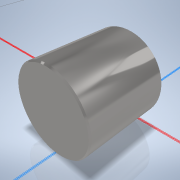
# Autodesk Inventor part: ciezarek
Saved by Autodesk Inventor 2021 (Build 250183000, 183)
## iProperties
Created: 2021-11-16
Part Number: ciezarek
Material: Stal nierdzewna 440C
Document SubType Name: Modeling
Designer: wojwo
Mass: 48.6178 g
Surface Area: 18.5509 cm^2
Volume: 6.27327 cm^3
Density: 7.75 g/cm^3
Appearance: Częściowo polerowana
Author: wojwo
Autodesk Inventor part; units mm, degrees
ref_plane "YZ Plane" through (0, 0, 0) normal (1, 0, 0) x (0, 1, 0)
ref_plane "XZ Plane" through (0, 0, 0) normal (0, 1, 0) x (-1, 0, 0)
ref_plane "XY Plane" through (0, 0, 0) normal (0, 0, 1) x (1, 0, 0)
sketch "Szkic1" plane through (0, 0, 0) normal (0, 0, 1) x (1, 0, 0)
  circle A0 centre (0, -7.5) radius 4.5 projected
  circle A1 centre (0, 0) radius 39.6 projected
  circle A2 centre (0, 7.5) radius 4.5 projected
  circle A3 centre (0, -7.5) radius 4.5 projected
  circle A4 centre (0, 0) radius 39.6 projected
  circle A5 centre (0, 7.5) radius 4.5 projected
  circle A6 centre (0, 20) radius 10
  point P0 (0, 0)
  dimension "d0" = 20
  dimension "d6" = 20
  constraints: 1 centre point
  measures "d0" diameter of A6
  measures "d6" distance of point (0, 0) A6.centre
extrude "Wyciągnięcie proste1" add sketch "Szkic1" along normal blind 20 contours A6 A2 | A2 A6 picked at (0.176, 10.6981) picked at (-0.2387, 23.9402)
chamfer "Faza1" distance 0.4 angle 45 2 edges at (-10, 20, 0) (-10, 20, 20)
